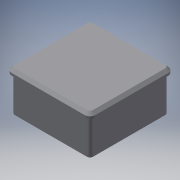
# Autodesk Inventor part: nút nhựa bịt hộp thép 60x60
Saved by Autodesk Inventor 2016 (Build 200138000, 138)
## iProperties
Created: 2018-11-14
Part Number: nút nhựa bịt hộp thép 60x60
Material: Generic
Document SubType Name: Modeling
Designer: hovm
Density: 1 g/cm^3
Appearance: Default
Author: hovm
Autodesk Inventor part; units mm, degrees
ref_plane "YZ Plane" through (0, 0, 0) normal (1, 0, 0) x (0, 1, 0)
ref_plane "XZ Plane" through (0, 0, 0) normal (0, 1, 0) x (-1, 0, 0)
ref_plane "XY Plane" through (0, 0, 0) normal (0, 0, 1) x (1, 0, 0)
sketch "Sketch1" plane through (0, 0, 0) normal (0, 0, 1) x (1, 0, 0)
  line L0 (26, 23) -> (-26, 23) projected
  arc A0 (-26, 23) -> (-28, 21) centre (-26, 21) ccw projected
  line L1 (-28, 21) -> (-28, -31) projected
  arc A1 (28, 21) -> (26, 23) centre (26, 21) ccw projected
  line L2 (28, -31) -> (28, 21) projected
  arc A2 (26, -33) -> (28, -31) centre (26, -31) ccw projected
  line L3 (-26, -33) -> (26, -33) projected
  arc A3 (-28, -31) -> (-26, -33) centre (-26, -31) ccw projected
  point P0 (0, 0)
extrude "Extrusion1" add sketch "Sketch1" against normal blind 30
sketch "Sketch2" plane through (0, 0, 0) normal (0, 0, 1) x (1, 0, 0)
  line L0 (26, 23) -> (-26, 23) projected
  arc A0 (28, 21) -> (26, 23) centre (26, 21) ccw projected
  line L1 (28, -31) -> (28, 21) projected
  arc A1 (26, -33) -> (28, -31) centre (26, -31) ccw projected
  line L2 (-26, -33) -> (26, -33) projected
  arc A2 (-28, -31) -> (-26, -33) centre (-26, -31) ccw projected
  line L3 (-28, 21) -> (-28, -31) projected
  arc A3 (-26, 23) -> (-28, 21) centre (-26, 21) ccw projected
  line L4 (-30, -31) -> (-30, 21) projected
  arc A4 (-30, -31) -> (-26, -35) centre (-26, -31) ccw projected
  line L5 (26, -35) -> (-26, -35) projected
  arc A5 (26, -35) -> (30, -31) centre (26, -31) ccw projected
  line L6 (30, 21) -> (30, -31) projected
  arc A6 (30, 21) -> (26, 25) centre (26, 21) ccw projected
  line L7 (-26, 25) -> (26, 25) projected
  arc A7 (-26, 25) -> (-30, 21) centre (-26, 21) ccw projected
  point P0 (0, 0)
extrude "Extrusion2" add sketch "Sketch2" along normal blind 4 contours A0 L1 A1 L2 A2 L3 A3 L0 | L4 A7 L7 A6 L6 A5 L5 A4
chamfer "Chamfer1" distance 1.5 angle 45 8 edges at (-30, -5, 4) (-28.8284, -33.8284, 4) (0, -35, 4) (28.8284, -33.8284, 4) (30, -5, 4) (28.8284, 23.8284, 4) (0, 25, 4) (-28.8284, 23.8284, 4)
chamfer "Chamfer2" distance 0.3 angle 45 8 edges at (-30, -5, 0) (-28.8284, 23.8284, 0) (0, 25, 0) (28.8284, 23.8284, 0) (30, -5, 0) (28.8284, -33.8284, 0) (0, -35, 0) (-28.8284, -33.8284, 0)
body "Solid1"
